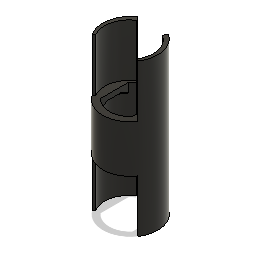
Battery_midspacer_2023.04.26 (Autodesk Fusion 360 design; units mm, degrees)
Autodesk Fusion 360 part; units mm, degrees
note: some values were not read from the file. Set by a fixed rule: which sketch regions a step uses.
sketch "Sketch1" plane through (0, 0, 0) normal (0, 1, 0) x (1, 0, 0)
  circle A0 centre (0, 0) radius 10.5
  circle A1 centre (0, -0.5) radius 9.25
  line L0 (8, 12) -> (0, 0)
  line L1 (0, 0) -> (-8, 12)
  line L2 (-12, -8) -> (0, 0)
  line L3 (0, 0) -> (12, -8)
  circle A2 centre (0, 0) radius 8
  line L4 (6, 8) -> (6, -7)
  line L5 (-6, 8) -> (-6, -7)
  point P0 (0, -0.5)
  dimension "d1" = 21
  dimension "d2" = 0.5
  dimension "d3" = 18.5
  dimension "d4" = 16
  constraint coincident A0.centre L0.end
  constraint vertical A0.centre A1.centre
  constraint coincident P0 A1.centre
  constraint vertical L4
  constraint vertical L5
  measures "d1" diameter of A0
  measures "d2" distance of A0.centre P0
  measures "d3" diameter of A1
  measures "d4" diameter of A2
extrude "Extrude1" add sketch "Sketch1" along normal blind 9 contours A0 A1 L0 L3 | A0 A1 L2 L3 | A0 A1 L1 L2 | A1 L0 A2 L4 | A1 L3 A2 L4 | A1 L2 L3 A2 | A1 L1 A2 L5 | A1 L2 A2 L5
extrude "Extrude2" add sketch "Sketch1" against normal blind 20 contours A0 A1 L0 L3 | A0 A1 L1 L2
extrude "Extrude3" add sketch "Sketch1" along normal blind 2 contours L3 A2 L4 | L3 A2 L4 | L2 A2 L5 | L2 A2 L5
chamfer "Chamfer1" distance 1.5 angle 45 1 edges at (8, 2, 0)
chamfer "Chamfer1" distance 1.5 angle 45 1 edges at (-8, 2, 0)
mirror "Mirror1" about plane through (0, 9, 0) normal (0, 1, 0) of bodies 1 merged
